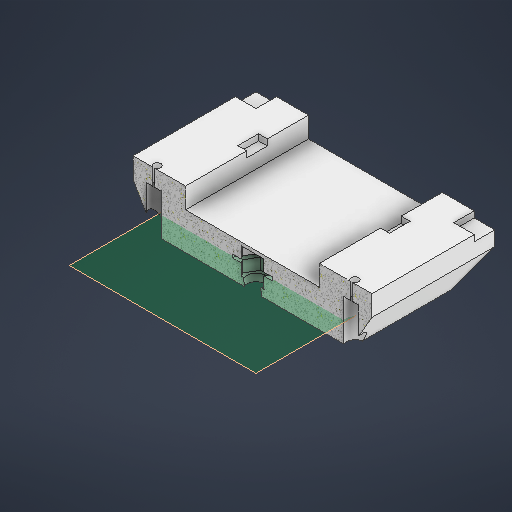
# Autodesk Inventor part: soporte_v1
Saved by Autodesk Inventor 2026 (Build 300175050, 175E)
## iProperties
Created: 2025-06-19
Part Number: soporte_v1
Material: Plástico ABS
Document SubType Name: Modeling
Designer: rodri
Density: 1.06 g/cm^3
Appearance: Suave - Blanco
Mass: 180.598 g
Surface Area: 321.427 cm^2
Volume: 170.376 cm^3
Author: rodri
## iProperties of the stored document soporte_v2_3DPrint.ipt
Created: 2025-07-11
Part Number: soporte_v2_3DPrint
Material: Genérico
Document SubType Name: Modeling
Designer: rodri
Density: 1 g/cm^3
Appearance: Valor por defecto
Author: rodri
Autodesk Inventor part; units mm, degrees
ref_plane "YZ Plane" through (0, 0, 0) normal (1, 0, 0) x (0, 1, 0)
ref_plane "XZ Plane" through (0, 0, 0) normal (0, 1, 0) x (-1, 0, 0)
ref_plane "XY Plane" through (0, 0, 0) normal (0, 0, 1) x (1, 0, 0)
sketch "Boceto31" plane through (0, 0, 0) normal (0, 1, 0) x (-1, 0, 0)
  line L0 (-58, 58) -> (58, 58)
  line L1 (58, 58) -> (58, -58)
  line L2 (58, -58) -> (-58, -58)
  line L3 (-58, -58) -> (-58, 58)
  line L4 (-58, 58) -> (58, -58) construction
  line L5 (58, 58) -> (-58, -58) construction
  line L6 (-32.5, 58) -> (32.5, 58)
  line L7 (32.5, 58) -> (32.5, -58)
  line L8 (32.5, -58) -> (-32.5, -58)
  line L9 (-32.5, -58) -> (-32.5, 58)
  line L10 (-32.5, 58) -> (32.5, -58) construction
  line L11 (32.5, 58) -> (-32.5, -58) construction
  line L12 (-48, 0) -> (48, 0) construction
  point P0 (0, 0)
  dimension "d155" = 116
  dimension "d156" = 116
  dimension "d157" = 65
  dimension "d158" = 96
  constraints: 26 end point, 5 midpoint, 4 parallel, 3 perpendicular, 2 horizontal, 1 point on line
  measures "d155" distance of L1.end L2.end
  measures "d156" distance of L0.end L1.end
  measures "d157" distance between parallel lines of L9 L7
  measures "d158" distance of L12.start L12.end
extrude "Extrusión10" add sketch "Boceto31" against normal blind 10 contours L0 L9 L2 L3 | L0 L1 L2 L7
sketch "Boceto32" plane through (0, -10, 0) normal (0, -1, 0) x (1, 0, 0)
  line L0 (-32.5, 58) -> (-58, 58) projected
  line L1 (58, -58) -> (58, 58) projected
  line L2 (-58, 58) -> (58, 58)
  line L3 (58, 58) -> (58, -58)
  line L4 (58, -58) -> (-58, -58)
  line L5 (-58, -58) -> (-58, 58)
  point P0 (0, 0)
  constraints: 8 end point, 2 parallel, 1 horizontal, 1 perpendicular
extrude "Extrusión11" add sketch "Boceto32" along normal blind 18 draft -30
hole "Agujero7" at (-48, 0, 0) at (48, 0, 0) direction (0, -1, 0) diameter 3.6 end through all clearance for "Tornillo para maquinaria de cabeza plana" size "M3" standard "Perfil M métrico ANSI"
ref_plane "Plano de trabajo10" through (0, -18, 0) normal (0, -1, 0) x (1, 0, 0)
sketch "Boceto33" plane through (0, -18, 0) normal (0, -1, 0) x (1, 0, 0)
  line L0 (6.4663, 0) -> (3.2332, -5.6)
  line L1 (3.2332, -5.6) -> (-3.2332, -5.6)
  line L2 (-3.2332, -5.6) -> (-6.4663, 0)
  line L3 (-6.4663, 0) -> (-3.2332, 5.6)
  line L4 (-3.2332, 5.6) -> (3.2332, 5.6)
  line L5 (3.2332, 5.6) -> (6.4663, 0)
  point P0 (0, 0)
  point P1 (0, 0)
  dimension "d212" = 11.2
  constraints: 12 end point, 1 coincident, 13 other
  measures "d212" distance between parallel lines of L2 L5
extrude "Extrusión12" cut sketch "Boceto33" along normal mid plane 12.8
sketch "Boceto34" plane through (0, -28, 0) normal (0, -1, 0) x (1, 0, 0)
  arc A0 (-47.6077, 1.7567) -> (-47.6077, -1.7567) centre (-48, 0) ccw projected
  circle A1 centre (-48, 0) radius 4
  line L0 (-17.8562, 0) -> (-10.0366, 0) construction
  circle A2 centre (48, 0) radius 4
  arc A3 (47.6077, -1.7567) -> (47.6077, 1.7567) centre (48, 0) ccw projected
  point P0 (0, 0)
  point P1 (0, 0)
  dimension "d194" = 8
  dimension "d197" = 96
  constraints: 2 centre point, 2 coincident, 2 end point, 2 horizontal, 2 other
  measures "d194" diameter of A1
  measures "d197" distance of A1.centre A2.centre
hole "Agujero9" at (0, -28, 0) direction (0, 1, 0) diameter 9 depth 3.6 clearance for "Perno de cabeza hexagonal" size "M8" standard "Perfil M métrico ANSI"
sketch "Boceto35" plane through (0, 0, 0) normal (0, 1, 0) x (1, 0, 0)
  line L0 (-58, -58) -> (-58, 58) projected
  line L1 (-58, 58) -> (-48, 58)
  line L2 (-48, 58) -> (-48, 48)
  line L3 (-48, 48) -> (-58, 48)
  line L4 (-58, 48) -> (-58, 58)
  line L5 (-32.5, 58) -> (-32.5, -58) projected
  line L6 (-32.5, 38) -> (-36.8198, 38)
  line L7 (-36.8198, 38) -> (-36.8198, 28)
  line L8 (-36.8198, 28) -> (-32.5, 28)
  line L9 (-32.5, 28) -> (-32.5, 38)
  line L10 (-32.5, 58) -> (-58, 58) projected
  point P0 (0, 0)
  dimension "d188" = 10
  dimension "d189" = 10
  dimension "d190" = 10
  dimension "d191" = 20
  constraints: 16 end point, 4 parallel, 2 horizontal, 2 perpendicular, 1 point on line
  measures "d188" distance of L2.end L3.end
  measures "d189" distance of L1.end L2.end
  measures "d190" distance of L6.end L7.end
  measures "d191" distance between parallel lines of L6 L10
extrude "Extrusión13" cut sketch "Boceto35" against normal blind 3
mirror "Simetría2" about plane through (0, 0, 0) normal (1, 0, 0) of "Extrusión13"
mirror "Simetría3" about plane through (0, 0, 0) normal (0, 0, 1) of "Extrusión13", "Simetría2"
extrude "Extrusión14" cut sketch "Boceto34" against normal blind 20
sketch "Boceto37" plane through (0, -18, 0) normal (0, -1, 0) x (1, 0, 0)
  circle A0 centre (0, 0) radius 9.75
  dimension "d209" = 19.5
  constraints: 1 centre point, 1 coincident
  measures "d209" diameter of A0
extrude "Extrusión16" cut sketch "Boceto37" along normal mid plane 1.64
